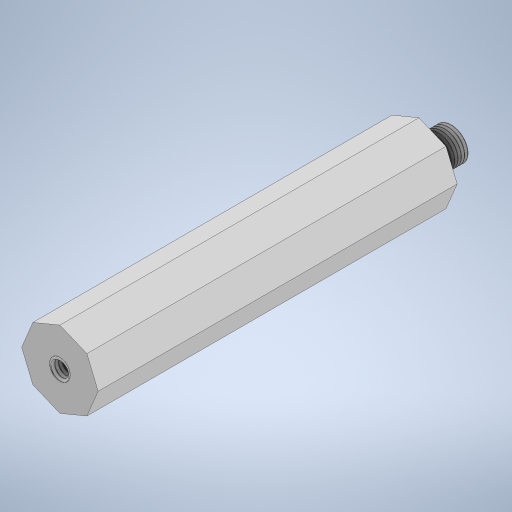
# Autodesk Inventor part: mark-10 adapter_modified
Saved by Autodesk Inventor 2024 (Build 280153000, 153)
## iProperties
Created: 2022-06-16
Part Number: mark-10 adapter_modified
Material: 일반
Document SubType Name: Modeling
Designer: Yeong Jae Park
Density: 1 g/cm^3
Appearance: 기본값
Author: Yeong Jae Park
Autodesk Inventor part; units mm, degrees
ref_plane "YZ Plane" through (0, 0, 0) normal (1, 0, 0) x (0, 1, 0)
ref_plane "XZ Plane" through (0, 0, 0) normal (0, 1, 0) x (-1, 0, 0)
ref_plane "XY Plane" through (0, 0, 0) normal (0, 0, 1) x (1, 0, 0)
sketch "스케치1" plane through (0, 0, 0) normal (0, 0, 1) x (1, 0, 0)
  circle A0 centre (0, 0) radius 6.35
  dimension "d0" = 12.7
  constraints: 1 centre point, 1 coincident
  measures "d0" diameter of A0
extrude "돌출1" add sketch "스케치1" along normal blind 10.16
sketch "스케치2" plane through (0, 0, 10.16) normal (0, 0, 1) x (1, 0, 0)
  circle A0 centre (0, 0) radius 6.35
  constraints: 1 centre point, 1 coincident
extrude "돌출2" add sketch "스케치2" along normal blind 139.7
thread "스레드1" size "1/2-20 UNF" class "2A" standard "ANSI Unified Screw Threads" length 12.7
sketch "스케치3" plane through (0, 0, 149.86) normal (0, 0, 1) x (1, 0, 0)
  circle A0 centre (0, 0) radius 3.9688
  dimension "d7" = 7.9375
  constraints: 1 centre point, 1 coincident
  measures "d7" diameter of A0
extrude "돌출3" cut sketch "스케치3" against normal blind 7.62
thread "스레드2" size "5/16-18 UNC" class "2B" standard "ANSI Unified Screw Threads" length 10.16
sketch "스케치4" plane through (0, 0, 149.86) normal (0, 0, 1) x (1, 0, 0)
  circle A0 centre (0, 0) radius 6.35 projected
  line L0 (0, 6.35) -> (0, -6.35) construction
  line L1 (-6.35, 0) -> (6.35, 0) construction
  line L2 (-6.35, 0) -> (-4.4901, 4.4901)
  line L3 (-4.4901, 4.4901) -> (0, 6.35)
  line L4 (0, 0) -> (-4.4901, 4.4901) construction
  line L5 (6.35, 0) -> (4.4901, 4.4901)
  line L6 (4.4901, 4.4901) -> (0, 6.35)
  line L7 (-6.35, 0) -> (-4.4901, -4.4901)
  line L8 (-4.4901, -4.4901) -> (0, -6.35)
  line L9 (4.4901, -4.4901) -> (0, -6.35)
  line L10 (6.35, 0) -> (4.4901, -4.4901)
  dimension "d12" = 45
  constraints: 22 end point, 5 point on circle, 4 midpoint, 3 symmetric about line, 1 horizontal, 1 vertical
  measures "d12" angle of L4 L1
extrude "돌출4" cut sketch "스케치4" against normal blind 12.7 contours L5 A0 | A0 L10 | L6 A0 | A0 L9 | L3 A0 | A0 L8 | L2 A0 | A0 L7
sketch "스케치5" plane through (0, 0, 149.86) normal (0, 0, 1) x (1, 0, 0)
  line L0 (4.4901, -4.4901) -> (6.35, 0) projected
  line L1 (6.35, 0) -> (4.4901, 4.4901) projected
  line L2 (4.4901, 4.4901) -> (0, 6.35) projected
  line L3 (0, 6.35) -> (-4.4901, 4.4901) projected
  line L4 (-4.4901, 4.4901) -> (-6.35, 0) projected
  line L5 (-6.35, 0) -> (-4.4901, -4.4901) projected
  line L6 (-4.4901, -4.4901) -> (0, -6.35) projected
  line L7 (0, -6.35) -> (4.4901, -4.4901) projected
  circle A0 centre (0, 0) radius 3.9687 projected
  line L8 (0, 14.5978) -> (10.3222, 10.3222)
  line L9 (10.3222, 10.3222) -> (14.5978, 0)
  line L10 (14.5978, 0) -> (10.3222, -10.3222)
  line L11 (10.3222, -10.3222) -> (0, -14.5978)
  line L12 (0, -14.5978) -> (-10.3222, -10.3222)
  line L13 (-10.3222, -10.3222) -> (-14.5978, 0)
  line L14 (-14.5978, 0) -> (-10.3222, 10.3222)
  line L15 (-10.3222, 10.3222) -> (0, 14.5978)
  dimension "d15" = 7.62
  constraints: 16 end point, 7 other
  measures "d15" distance between parallel lines of L2 L8
extrude "돌출5" add sketch "스케치5" against normal blind 137.16 contours L8 L9 L10 L11 L12 L13 L14 L15
sketch "스케치7" plane through (0, 0, 0) normal (1, 0, 0) x (0, 1, 0)
  line L0 (6.35, 0) -> (6.35, 12.7)
  line L1 (6.35, 12.7) -> (5.4083, 12.7)
  line L2 (5.4083, 12.7) -> (5.4083, 0)
  line L3 (5.4083, 0) -> (6.35, 0)
  line L4 (0, -31.6339) -> (0, 180.109) projected
  constraints: 8 end point
revolve "회전1" cut sketch "스케치7" angle 360 about axis through (0, 0, 0) along (0, 0, 1)
sketch "스케치8" plane through (0, 0, 0) normal (1, 0, 0) x (0, 1, 0)
  line L0 (6.35, 0) -> (6.35, 12.7)
  line L1 (6.35, 12.7) -> (5.4083, 12.7)
  line L2 (5.4083, 12.7) -> (5.4083, 0)
  line L3 (5.4083, 0) -> (6.35, 0)
  line L4 (0, -31.6339) -> (0, 180.109) projected
  constraints: 8 end point
revolve "회전2" add sketch "스케치8" angle 360 about axis through (0, 0, 0) along (0, 0, 1) separate body
sketch "스케치6" plane through (0, 0, 0) normal (-1, 0, 0) x (0, 0, 1)
  line L0 (-0.7409, -5.4727) -> (-0.6351, -5.4727) construction
  line L1 (0.1057, -6.2859) -> (-0.0001, -6.4893) construction
  line L2 (-1.2701, -6.4893) -> (-1.3759, -6.2859) construction
  line L3 (-0.5293, -5.4727) -> (-0.6351, -5.2694) construction
  line L4 (-0.6351, -5.2694) -> (-0.7409, -5.4727) construction
  line L5 (-1.2701, -6.4893) -> (-1.1643, -6.2859) construction
  line L6 (-0.5293, -5.4727) -> (-0.1059, -6.2859)
  line L7 (-1.3759, -6.2859) -> (-1.1643, -6.2859) construction
  arc A0 (-1.3759, -6.2859) -> (-1.2701, -6.3502) centre (-1.2701, -6.2309) ccw construction
  line L8 (0.1057, -6.2859) -> (-0.1059, -6.2859) construction
  line L9 (-1.2701, -6.4893) -> (-1.2701, -6.2859) construction
  line L10 (-0.0001, -6.4893) -> (-0.0001, -6.2859) construction
  line L11 (-0.6351, -5.2694) -> (-0.6351, -5.4085) construction
  line L12 (-1.2701, -6.3502) -> (-0.0001, -6.3502)
  arc A1 (-1.2701, -6.3502) -> (-1.1643, -6.2859) centre (-1.2701, -6.2309) ccw
  line L13 (-0.1059, -6.2859) -> (-0.0001, -6.4893) construction
  line L14 (-1.1643, -6.2859) -> (-0.7409, -5.4727)
  line L15 (-0.0001, -0.0002) -> (-0.0001, 0.0177)
  line L16 (-0.0001, 0.0177) -> (-0.0001, -0.0002)
  line L17 (-0.0001, -0.0002) -> (0.0334, -0.0002)
  arc A2 (-0.1059, -6.2859) -> (-0.0001, -6.3502) centre (-0.0001, -6.2309) ccw
  arc A3 (-0.0001, -6.3502) -> (0.1057, -6.2859) centre (-0.0001, -6.2309) ccw construction
  arc A4 (-0.6351, -5.4085) -> (-0.7409, -5.4727) centre (-0.6351, -5.5278) ccw
  arc A5 (-0.5293, -5.4727) -> (-0.6351, -5.4085) centre (-0.6351, -5.5278) ccw
  line L18 (-0.6351, -5.4085) -> (-0.6351, -5.4727) construction
  line L19 (-0.6351, -5.4727) -> (-0.5293, -5.4727) construction
  dimension "d18" = 55
  dimension "d19" = 0.2033
  dimension "d20" = 0.2033
  dimension "d23" = 1.27
  constraints: 40 end point, 12 point on circle, 10 parallel, 8 tangent, 7 collinear, 6 centre point, 2 midpoint, 2 point on line, 1 horizontal, 1 perpendicular, 5 other
  measures "d18" angle of L6 L14
  measures "d19" distance of L3.end L0.end
  measures "d20" distance of L1.end L10.end
  measures "d23" distance from line of L1.end L9
coil "코일1" sketch "스케치6" operation cut axis through (0, 0, 0) along (0, 0, 1) pitch 1.2713 turns 11.988012 hand right bodies 2
sketch "스케치10" plane through (0, 0, 149.86) normal (-1, 0, 0) x (0, 1, 0)
  line L0 (3.9688, 0) -> (3.9688, 10.16)
  line L1 (3.9688, 10.16) -> (2.9225, 10.16)
  line L2 (2.9225, 10.16) -> (2.9225, 0)
  line L3 (2.9225, 0) -> (3.9688, 0)
  line L4 (0, -31.9032) -> (0, 180.6478) projected
  constraints: 8 end point
revolve "회전3" add sketch "스케치10" angle 360 about axis through (0, 0, 149.86) along (0, 0, -1) separate body
sketch "스케치9" plane through (0, 3.9688, 149.86) normal (1, 0, 0) x (0, 0, -1)
  line L0 (-0.8233, -0.0715) -> (-0.7057, -0.0715) construction
  line L1 (0.1175, -0.9751) -> (-0.0001, -1.201) construction
  line L2 (-1.4112, -1.201) -> (-1.5288, -0.9751) construction
  line L3 (-0.5881, -0.0715) -> (-0.7057, 0.1544) construction
  line L4 (-0.7057, 0.1544) -> (-0.8233, -0.0715) construction
  line L5 (-1.4112, -1.201) -> (-1.2936, -0.9751) construction
  line L6 (-0.5881, -0.0715) -> (-0.1177, -0.9751)
  line L7 (-1.5288, -0.9751) -> (-1.2936, -0.9751) construction
  arc A0 (-1.5288, -0.9751) -> (-1.4112, -1.0465) centre (-1.4112, -0.9139) ccw construction
  line L8 (0.1175, -0.9751) -> (-0.1177, -0.9751) construction
  line L9 (-1.4112, -1.201) -> (-1.4112, -0.9751) construction
  line L10 (-0.0001, -1.201) -> (-0.0001, -0.9751) construction
  line L11 (-0.7057, 0.1544) -> (-0.7057, -0.0002) construction
  line L12 (-1.4112, -1.0465) -> (-0.0001, -1.0465)
  arc A1 (-1.4112, -1.0465) -> (-1.2936, -0.9751) centre (-1.4112, -0.9139) ccw
  line L13 (-0.1177, -0.9751) -> (-0.0001, -1.201) construction
  line L14 (-1.2936, -0.9751) -> (-0.8233, -0.0715)
  line L15 (-0.0001, -0.0002) -> (-0.0001, 0.0177)
  line L16 (-0.0001, 0.0177) -> (-0.0001, -0.0002)
  line L17 (-0.0001, -0.0002) -> (0.0334, -0.0002)
  arc A2 (-0.1177, -0.9751) -> (-0.0001, -1.0465) centre (-0.0001, -0.9139) ccw
  arc A3 (-0.0001, -1.0465) -> (0.1175, -0.9751) centre (-0.0001, -0.9139) ccw construction
  arc A4 (-0.7057, -0.0002) -> (-0.8233, -0.0715) centre (-0.7057, -0.1327) ccw
  arc A5 (-0.5881, -0.0715) -> (-0.7057, -0.0002) centre (-0.7057, -0.1327) ccw
  line L18 (-0.7057, -0.0002) -> (-0.7057, -0.0715) construction
  line L19 (-0.7057, -0.0715) -> (-0.5881, -0.0715) construction
  dimension "d37" = 55
  dimension "d38" = 0.2259
  dimension "d39" = 0.2259
  dimension "d42" = 1.4111
  constraints: 40 end point, 12 point on circle, 10 parallel, 9 tangent, 7 collinear, 6 centre point, 2 midpoint, 2 point on line, 1 horizontal, 1 perpendicular, 4 other
  measures "d37" angle of L6 L14
  measures "d38" distance of L3.end L0.end
  measures "d39" distance of L1.end L10.end
  measures "d42" distance from line of L1.end L9
coil "코일2" sketch "스케치9" operation cut axis through (0, 0, 149.86) along (0, 0, -1) pitch 1.4125 turns 9.190809 hand right bodies 3
equation "\"d18\" = d25"
equation "\"d37\" = d44"
equation "\"d25\" = 55deg"
equation "\"d44\" = 55deg"
